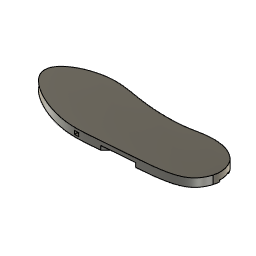
Smart foot brace v3 (Autodesk Fusion 360 design; units mm, degrees)
Autodesk Fusion 360 part; units mm, degrees
sketch "Schizzo2" plane through (0, 0, 0) normal (0, 0, 1) x (1, 0, 0)
  line L0 (-49.9969, 3.1408) -> (-49.9969, -77.002)
  line L1 (269.0032, -13.0421) -> (245.6537, -14.8322)
  line L2 (251.2577, -31.5554) -> (270.315, -30.0944)
  line L3 (270.315, -30.0944) -> (269.0032, -13.0421)
  spline S0 degree 5 poles (239.6431, -39.0842) (239.008, -40.9338) (237.6138, -44.5456) (235.154, -49.7023) (230.6516, -55.9329) (221.1905, -62.1637) (206.5229, -66.4683) (188.36, -69.1663) (168.6133, -70.9116) (148.4991, -72.3278) (128.8774, -73.8918) (110.0255, -75.6871) (91.7256, -77.2705) (73.0453, -77.351) (52.5897, -73.8128) (31.6095, -66.6537) (12.3777, -56.7145) (-2.2618, -45.4213) (-9.8521, -34.1339) (-8.9725, -23.6462) (-0.2666, -13.6017) (14.0848, -4.9823) (31.2393, 1.0769) (48.4813, 3.7209) (63.9221, 3.1001) (77.5489, 1.0443) (90.8033, -1.4303) (105.5547, -3.5848) (122.705, -4.9647) (142.1637, -5.3299) (159.3113, -4.3034) (172.1696, -2.1405) (182.8837, 0.235) (193.8253, 1.7835) (206.3024, 1.6151) (216.9338, -0.4964) (223.8154, -3.6611) (228.407, -6.7709) (231.3167, -9.1532) (232.7333, -10.4216) knots 0 0 0 0 0 0 0.028571 0.057143 0.085714 0.114286 0.142857 0.171429 0.2 0.228571 0.257143 0.285714 0.314286 0.342857 0.371429 0.4 0.428571 0.457143 0.485714 0.514286 0.542857 0.571429 0.6 0.628571 0.657143 0.685714 0.714286 0.742857 0.771429 0.8 0.828571 0.857143 0.885714 0.914286 0.942857 0.971429 1 1 1 1 1 1
  line L4 (247.2731, -16.8633) -> (232.013, -61.305)
  line L5 (235.4873, -58.3623) -> (184.5271, -71.6971)
  line L6 (112.4168, -77.0193) -> (57.595, -77.0134)
  line L7 (-8.4307, -44.1652) -> (-8.4277, -15.72)
  line L8 (26.8163, 3.1326) -> (81.9854, 3.1268)
  line L9 (104.9495, -5.3071) -> (173.0776, -4.7372)
  line L10 (173.2743, 1.9517) -> (226.7543, 0.991)
  line L11 (214.0903, 6.2711) -> (251.3764, -27.1143)
  spline S1 degree 5 poles (239.6431, -39.0842) (239.8525, -38.4743) (240.3443, -37.3331) (241.301, -35.8564) (242.9551, -34.3027) (245.4512, -32.8887) (247.6708, -32.1165) (249.4288, -31.7477) (250.6413, -31.6027) (251.2577, -31.5554) knots 0 0 0 0 0 0 0.2 0.4 0.6 0.8 1 1 1 1 1 1
  spline S2 degree 5 poles (232.7333, -10.4216) (233.164, -10.8072) (234.0487, -11.5321) (235.446, -12.4805) (237.4316, -13.4935) (240.0595, -14.3948) (242.2482, -14.8107) (243.9334, -14.9127) (245.0769, -14.8765) (245.6537, -14.8322) knots 0 0 0 0 0 0 0.2 0.4 0.6 0.8 1 1 1 1 1 1
  line L12 (-8.4292, -101.5202) -> (241.5708, -101.5202)
  line L13 (269.9236, -11.9686) -> (245.5773, -13.8352)
  spline S3 degree 3 poles (233.4004, -9.6766) (235.2721, -11.3525) (237.4456, -12.4757) (239.7715, -13.1715) (241.6374, -13.7297) (243.5687, -13.9891) (245.5773, -13.8352) knots 0 0 0 0 0.554866 0.554866 0.554866 1 1 1 1
  spline S4 degree 3 poles (240.5888, -39.4089) (239.2288, -43.3698) (237.586, -47.1235) (235.258, -50.5942) (233.0296, -53.9163) (230.1256, -56.9559) (226.1195, -59.5307) (222.5382, -61.8324) (218.0521, -63.7558) (212.7264, -65.3147) (204.0376, -67.858) (193.2175, -69.4408) (181.8239, -70.6189) (171.6726, -71.6685) (161.0707, -72.4189) (150.6531, -73.2094) (141.2105, -73.9259) (131.9202, -74.686) (122.8812, -75.4938) (114.5446, -76.2388) (106.4233, -77.0328) (98.2848, -77.5487) (90.3505, -78.0515) (82.3633, -78.2665) (73.9671, -77.5846) (66.6167, -76.9877) (58.9395, -75.6792) (51.1766, -73.6098) (41.5761, -71.0505) (31.86, -67.3391) (23.0777, -62.9007) (14.0271, -58.3266) (6.0213, -53.0215) (0.2781, -47.5919) (-4.7696, -42.8201) (-8.0755, -37.953) (-9.0908, -33.1359) (-9.8586, -29.4927) (-9.2793, -25.8888) (-7.517, -22.488) (-4.7337, -17.1171) (0.9259, -12.1616) (8.0905, -7.9878) (14.6953, -4.1401) (22.5473, -1.0036) (30.4783, 1.0609) (36.8948, 2.7312) (43.3496, 3.689) (49.4389, 4.0032) (55.9944, 4.3414) (62.1106, 3.9625) (67.845, 3.3046) (75.3924, 2.4387) (82.3167, 1.1103) (89.6988, -0.1009) (95.7767, -1.098) (102.2122, -2.0254) (109.3408, -2.7161) (114.6842, -3.2339) (120.4332, -3.6238) (126.4033, -3.8401) (133.1258, -4.0837) (140.0715, -4.0995) (146.4427, -3.8471) (151.9175, -3.6301) (156.9467, -3.2154) (161.4118, -2.663) (169.3887, -1.6762) (175.6132, -0.2481) (181.8504, 0.8561) (185.556, 1.5122) (189.2963, 2.0447) (193.2224, 2.3041) (198.2672, 2.6374) (203.5926, 2.5112) (208.4512, 1.8288) (213.3705, 1.1379) (217.7793, -0.1161) (221.6768, -1.8868) (226.0615, -3.8789) (229.8582, -6.505) (233.4004, -9.6766) knots 0 0 0 0 0.03616105 0.03616105 0.03616105 0.07077455 0.07077455 0.07077455 0.10171712 0.10171712 0.10171712 0.15219932 0.15219932 0.15219932 0.19717723 0.19717723 0.19717723 0.23794526 0.23794526 0.23794526 0.27554534 0.27554534 0.27554534 0.31220121 0.31220121 0.31220121 0.34429112 0.34429112 0.34429112 0.38397767 0.38397767 0.38397767 0.42487674 0.42487674 0.42487674 0.46082195 0.46082195 0.46082195 0.48800841 0.48800841 0.48800841 0.53094375 0.53094375 0.53094375 0.57052484 0.57052484 0.57052484 0.60254726 0.60254726 0.60254726 0.63702043 0.63702043 0.63702043 0.68239288 0.68239288 0.68239288 0.71974977 0.71974977 0.71974977 0.74775154 0.74775154 0.74775154 0.77928259 0.77928259 0.77928259 0.80637744 0.80637744 0.80637744 0.85478308 0.85478308 0.85478308 0.88354135 0.88354135 0.88354135 0.92049365 0.92049365 0.92049365 0.95790815 0.95790815 0.95790815 1 1 1 1
  spline S5 degree 3 poles (240.5888, -39.4089) (241.3059, -37.3208) (242.5674, -35.9265) (244.2133, -34.8517) (245.985, -33.6946) (248.1383, -32.9425) (250.4491, -32.6435) (250.7409, -32.6057) (251.0358, -32.5753) (251.3342, -32.5525) knots 0 0 0 0 0.452012 0.452012 0.452012 0.938578 0.938578 0.938578 1 1 1 1
  line L14 (251.3342, -32.5525) -> (271.3887, -31.015)
  line L15 (271.3887, -31.015) -> (269.9236, -11.9686)
  spline S6 degree 3 poles (243.4498, -40.3145) (243.442, -40.3374) (243.4341, -40.3603) (243.4262, -40.3832) (242.0634, -44.3523) (240.3996, -48.2035) (238.0265, -51.8462) (235.6744, -55.4566) (232.5576, -58.8379) (228.3332, -61.6662) (224.4374, -64.2746) (219.6477, -66.3777) (214.0375, -68.0553) (204.0845, -71.0316) (191.6967, -72.693) (178.8207, -73.9334) (168.6765, -74.9106) (158.2217, -75.637) (148.0073, -76.4198) (138.7072, -77.1325) (129.5865, -77.902) (120.6933, -78.7021) (112.4086, -79.4474) (104.2918, -80.2322) (96.0615, -80.6859) (88.7013, -81.0916) (81.1926, -81.2067) (73.3032, -80.5399) (65.6523, -79.8932) (57.6694, -78.4919) (49.6214, -76.2976) (39.5371, -73.5481) (29.3854, -69.5745) (20.2705, -64.8326) (11.3691, -60.2017) (3.5101, -54.8955) (-2.2653, -49.3107) (-6.7675, -44.9572) (-10.0656, -40.3962) (-11.5628, -35.5397) (-11.7947, -34.7875) (-11.9824, -34.0288) (-12.123, -33.2646) (-12.8162, -29.4949) (-12.2823, -25.6931) (-10.7144, -22.2104) (-8.3374, -16.9306) (-3.8076, -12.3656) (1.8783, -8.3928) (2.4386, -8.0013) (3.0106, -7.6156) (3.5933, -7.2357) (10.8043, -2.5345) (19.6906, 1.2501) (28.7492, 3.7056) (35.3784, 5.5025) (42.0699, 6.5654) (48.4105, 6.9501) (55.1171, 7.3571) (61.376, 7.0246) (67.1852, 6.3967) (74.9752, 5.5546) (82.0081, 4.2133) (89.3533, 2.9966) (95.368, 2.0003) (101.6744, 1.0688) (108.6597, 0.3657) (113.8765, -0.1593) (119.4922, -0.5623) (125.3539, -0.7978) (132.0277, -1.066) (138.9779, -1.1101) (145.3609, -0.8855) (150.7837, -0.6946) (155.782, -0.3097) (160.2056, 0.2129) (167.2628, 1.0468) (172.9356, 2.2385) (178.5539, 3.3007) (182.5227, 4.0511) (186.4973, 4.7256) (190.7246, 5.1154) (195.4849, 5.5543) (200.543, 5.6207) (205.4013, 5.1935) (210.2533, 4.7669) (214.8072, 3.8537) (218.9098, 2.4397) (225.3474, 0.2209) (230.6534, -3.1902) (235.4016, -7.4416) (235.428, -7.4652) (235.4544, -7.4889) (235.4808, -7.5125) knots -0.00020611 -0.00020611 -0.00020611 -0.00020611 0 0 0 0.03482635 0.03482635 0.03482635 0.06918618 0.06918618 0.06918618 0.10083869 0.10083869 0.10083869 0.15703627 0.15703627 0.15703627 0.20132062 0.20132062 0.20132062 0.24164672 0.24164672 0.24164672 0.27922087 0.27922087 0.27922087 0.31279914 0.31279914 0.31279914 0.34534649 0.34534649 0.34534649 0.38613373 0.38613373 0.38613373 0.4259753 0.4259753 0.4259753 0.45704046 0.45704046 0.45704046 0.46185185 0.46185185 0.46185185 0.4854789 0.4854789 0.4854789 0.52150819 0.52150819 0.52150819 0.52505893 0.52505893 0.52505893 0.56895312 0.56895312 0.56895312 0.60106672 0.60106672 0.60106672 0.63505887 0.63505887 0.63505887 0.68067651 0.68067651 0.68067651 0.71802793 0.71802793 0.71802793 0.74591886 0.74591886 0.74591886 0.777679 0.777679 0.777679 0.80466247 0.80466247 0.80466247 0.8477088 0.8477088 0.8477088 0.87807551 0.87807551 0.87807551 0.91224796 0.91224796 0.91224796 0.94637208 0.94637208 0.94637208 1 1 1 1.0003083 1.0003083 1.0003083 1.0003083
  arc A0 (243.4498, -40.3145) -> (235.4808, -7.5125) centre (209.2626, -31.2511) ccw
  point P0 (-8.4292, -29.9426)
  point P1 (54.4009, 3.1297)
  point P2 (139.0136, -5.0221)
  point P3 (200.0143, 1.4714)
  point P4 (85.0059, -77.0164)
  point P5 (210.0072, -65.0297)
  point P6 (85.0059, -77.0164)
  point P7 (85.0059, -81.0152)
  dimension "d6" = 80.1428
  dimension "d10" = 250
  dimension "d15" = 1
  constraint parallel L1 L2
  constraint midpoint S0.start L4
  constraint midpoint P5 L5
  constraint midpoint P6 L6
  constraint midpoint P0 L7
  constraint midpoint P1 L8
  constraint midpoint P2 L9
  constraint midpoint P3 L10
  constraint midpoint S0.end L11
  constraint horizontal L12
  constraint vertical L0
  constraint coincident P6 P4
  constraint coincident S6 P7
  measures "d6" distance of L0.start L0.end
  measures "d10" distance of L12.start L12.end
extrude "Estrusione3" add sketch "Schizzo2" against normal blind 12 contours L11 S2 A0 | L11 S2 S3 S4 A0 | S0 L4 L11 A0 | S0 L10 L11 S4 | L10 L11 S3 S4 S6 A0 | L4 S1 S4 S5 A0 | L4 S1 A0 | S0 L8 L10 S4 | L10 S4 | L10 L11 S4 | S0 L4 L5 S4 | L4 S4 S5 S6 A0 | L7 L10 L11 S4 S6 | L10 L11 S6 | S0 L5 L6 S4 | L5 S4 | L4 L5 S4 S6 | S0 L7 L8 S4 | L8 S4 | S0 L6 L7 S4 | L6 S4 | L5 L7 S4 S6 | L7 S4 | L7 S4 S6
extrude "Estrusione4" [suppressed]
ref_plane "Piano di lavoro1" through (85.0059, -81.0152, 0) normal (-0.000242, -1, 0) x (1, -0.000242, 0)
sketch "Schizzo5" plane through (85.0059, -81.0152, 0) normal (-0.000242, -1, 0) x (1, -0.000242, 0)
  line L0 (158.4341, -12) -> (-97.4394, -12)
  line L1 (-93.4302, 0) -> (156.5698, 0)
  line L2 (6.35, -9.7) -> (-6.35, -9.7)
  line L3 (-6.35, -9.7) -> (-6.35, -3)
  line L4 (-6.35, -3) -> (6.35, -3)
  line L5 (6.35, -3) -> (6.35, -9.7)
  line L6 (3, -8.85) -> (-3, -8.85)
  line L7 (-3, -8.85) -> (-3, -3.85)
  line L8 (-3, -3.85) -> (3, -3.85)
  line L9 (3, -3.85) -> (3, -8.85)
  point P0 (1, -1)
  dimension "d56" = 3
  dimension "d57" = 12.7
  dimension "d58" = 6.7
  dimension "d59" = 6
  dimension "d60" = 5
  dimension "d62" = 0.85
  dimension "d63" = 3.35
  constraint horizontal L2
  constraint vertical L3
  constraint horizontal L4
  constraint vertical L5
  constraint horizontal L6
  constraint vertical L7
  constraint horizontal L8
  constraint vertical L9
  measures "d56" distance of L1 L4
  measures "d57" distance of L3.end L4.end
  measures "d58" distance of L2.start L4.end
  measures "d59" distance of L6.start L6.end
  measures "d60" distance of L6 L8
  measures "d62" distance of L2 L6
  measures "d63" distance of L3 L7
extrude "Estrusione11" cut sketch "Schizzo5" against normal blind 18.5 contours L6 L7 L8 L9
extrude "Estrusione12" cut sketch "Schizzo5" against normal blind 14.5 from surface at -4
extrude "Estrusione13" cut 1 faces at (82.8925, -67.348, -3) along direction (0, 0, -1) blind 20
sketch "Schizzo3" plane through (0, 0, -12) normal (0, 0, -1) x (1, 0, 0)
  arc A0 (235.4808, 7.5125) -> (243.4498, 40.3145) centre (209.2626, 31.2511) ccw
  spline S0 degree 3 poles (243.4498, 40.3145) (243.442, 40.3374) (243.4341, 40.3603) (243.4262, 40.3832) (242.0634, 44.3523) (240.3996, 48.2035) (238.0265, 51.8462) (235.6744, 55.4566) (232.5576, 58.8379) (228.3332, 61.6662) (224.4374, 64.2746) (219.6477, 66.3777) (214.0375, 68.0553) (204.0845, 71.0316) (191.6967, 72.693) (178.8207, 73.9334) (168.6765, 74.9106) (158.2217, 75.637) (148.0073, 76.4198) (138.7072, 77.1325) (129.5865, 77.902) (120.6933, 78.7021) (112.4086, 79.4474) (104.2918, 80.2322) (96.0615, 80.6859) (88.7013, 81.0916) (81.1926, 81.2067) (73.3032, 80.5399) (65.6523, 79.8932) (57.6694, 78.4919) (49.6214, 76.2976) (39.5371, 73.5481) (29.3854, 69.5745) (20.2705, 64.8326) (11.3691, 60.2017) (3.5101, 54.8955) (-2.2653, 49.3107) (-6.7675, 44.9572) (-10.0656, 40.3962) (-11.5628, 35.5397) (-11.7947, 34.7875) (-11.9824, 34.0288) (-12.123, 33.2646) (-12.8162, 29.4949) (-12.2823, 25.6931) (-10.7144, 22.2104) (-8.3374, 16.9306) (-3.8076, 12.3656) (1.8783, 8.3928) (2.4386, 8.0013) (3.0106, 7.6156) (3.5933, 7.2357) (10.8043, 2.5345) (19.6906, -1.2501) (28.7492, -3.7056) (35.3784, -5.5025) (42.0699, -6.5654) (48.4105, -6.9501) (55.1171, -7.3571) (61.376, -7.0246) (67.1852, -6.3967) (74.9752, -5.5546) (82.0081, -4.2133) (89.3533, -2.9966) (95.368, -2.0003) (101.6744, -1.0688) (108.6597, -0.3657) (113.8765, 0.1593) (119.4922, 0.5623) (125.3539, 0.7978) (132.0277, 1.066) (138.9779, 1.1101) (145.3609, 0.8855) (150.7837, 0.6946) (155.782, 0.3097) (160.2056, -0.2129) (167.2628, -1.0468) (172.9356, -2.2385) (178.5539, -3.3007) (182.5227, -4.0511) (186.4973, -4.7256) (190.7246, -5.1154) (195.4849, -5.5543) (200.543, -5.6207) (205.4013, -5.1935) (210.2533, -4.7669) (214.8072, -3.8537) (218.9098, -2.4397) (225.3474, -0.2209) (230.6534, 3.1902) (235.4016, 7.4416) (235.428, 7.4652) (235.4544, 7.4889) (235.4808, 7.5125) knots -0.00020611 -0.00020611 -0.00020611 -0.00020611 0 0 0 0.03482635 0.03482635 0.03482635 0.06918618 0.06918618 0.06918618 0.10083869 0.10083869 0.10083869 0.15703627 0.15703627 0.15703627 0.20132062 0.20132062 0.20132062 0.24164672 0.24164672 0.24164672 0.27922087 0.27922087 0.27922087 0.31279914 0.31279914 0.31279914 0.34534649 0.34534649 0.34534649 0.38613373 0.38613373 0.38613373 0.4259753 0.4259753 0.4259753 0.45704046 0.45704046 0.45704046 0.46185185 0.46185185 0.46185185 0.4854789 0.4854789 0.4854789 0.52150819 0.52150819 0.52150819 0.52505893 0.52505893 0.52505893 0.56895312 0.56895312 0.56895312 0.60106672 0.60106672 0.60106672 0.63505887 0.63505887 0.63505887 0.68067651 0.68067651 0.68067651 0.71802793 0.71802793 0.71802793 0.74591886 0.74591886 0.74591886 0.777679 0.777679 0.777679 0.80466247 0.80466247 0.80466247 0.8477088 0.8477088 0.8477088 0.87807551 0.87807551 0.87807551 0.91224796 0.91224796 0.91224796 0.94637208 0.94637208 0.94637208 1 1 1 1.0003083 1.0003083 1.0003083 1.0003083
  line L0 (-9.0133, 39.7235) -> (19.2267, 39.7235)
  line L1 (19.2267, 39.7235) -> (19.2267, 20.4235)
  line L2 (19.2267, 20.4235) -> (-9.0133, 20.4235)
  line L3 (-9.0133, 20.4235) -> (-9.0133, 39.7235)
  line L4 (-1.0133, 25.8735) -> (-17.0133, 25.8735)
  line L5 (-17.0133, 25.8735) -> (-17.0133, 34.2735)
  line L6 (-17.0133, 34.2735) -> (-1.0133, 34.2735)
  line L7 (-1.0133, 34.2735) -> (-1.0133, 25.8735)
  line L8 (-1.0133, 25.8735) -> (-17.0133, 34.2735) construction
  line L9 (-17.0133, 25.8735) -> (-1.0133, 34.2735) construction
  line L10 (73.2267, 49.9714) -> (92.2267, 49.9714)
  line L11 (92.2267, 49.9714) -> (92.2267, 17.9714)
  line L12 (92.2267, 17.9714) -> (73.2267, 17.9714)
  line L13 (73.2267, 17.9714) -> (73.2267, 49.9714)
  line L14 (19.2267, 49.9714) -> (73.2267, 49.9714)
  line L15 (73.2267, 49.9714) -> (73.2267, 13.9714)
  line L16 (73.2267, 13.9714) -> (19.2267, 13.9714)
  line L17 (19.2267, 13.9714) -> (19.2267, 49.9714)
  line L18 (92.2267, 49.9714) -> (119.6267, 49.9714)
  line L19 (119.6267, 49.9714) -> (119.6267, 24.5714)
  line L20 (119.6267, 24.5714) -> (92.2267, 24.5714)
  line L21 (92.2267, 24.5714) -> (92.2267, 49.9714)
  line L22 (122.6267, 61.7471) -> (164.6267, 61.7471)
  line L23 (164.6267, 61.7471) -> (164.6267, 5.6113)
  line L24 (164.6267, 5.6113) -> (122.6267, 5.6113)
  line L25 (122.6267, 5.6113) -> (122.6267, 61.7471)
  line L26 (251.2577, 31.5554) -> (270.315, 30.0944)
  line L27 (270.315, 30.0944) -> (269.0032, 13.0421)
  line L28 (269.0032, 13.0421) -> (245.6537, 14.8322)
  line L29 (270.315, 30.0944) -> (269.0032, 13.0421)
  line L30 (269.0032, 13.0421) -> (209.18, 17.6439)
  line L31 (209.18, 17.6439) -> (210.4917, 34.6962)
  line L32 (210.4917, 34.6962) -> (270.315, 30.0944)
  line L33 (91.3569, 77.0167) -> (91.3604, 62.5167)
  line L34 (91.3604, 62.5167) -> (78.6604, 62.5136)
  line L35 (78.6604, 62.5136) -> (78.6569, 77.0136)
  line L36 (78.6569, 77.0136) -> (91.3569, 77.0167)
  line L37 (122.6267, 59.9714) -> (19.2267, 59.9714)
  line L38 (19.2267, 59.9714) -> (19.2267, 49.9714)
  line L39 (19.2267, 49.9714) -> (122.6267, 49.9714)
  line L40 (19.2267, 49.9714) -> (24.2267, 49.9714)
  line L41 (92.2267, 17.9714) -> (74.7267, 17.9714)
  line L42 (91.3604, 62.5167) -> (78.6619, 62.5167)
  line L43 (78.6619, 62.5167) -> (78.6619, 59.9714)
  line L44 (78.6619, 59.9714) -> (91.3604, 59.9714)
  line L45 (91.3604, 59.9714) -> (91.3604, 62.5167)
  line L46 (164.6267, 61.7471) -> (217.4262, 61.7471)
  line L47 (217.4262, 61.7471) -> (217.4262, 3.1169)
  line L48 (164.6267, 5.6113) -> (164.6267, 61.7471)
  spline S1 degree 5 poles (217.4262, 61.7471) (218.0377, 61.7142) (219.4226, 61.5343) (221.9857, 60.9195) (226.1571, 59.1373) (231.456, 53.9479) (235.4591, 45.0282) (236.9817, 32.4295) (235.4708, 19.7987) (231.4862, 10.8184) (226.2021, 5.5804) (222.0289, 3.8067) (219.4504, 3.2419) (218.0481, 3.1169) (217.4262, 3.1169) knots 0 0 0 0 0 0 0.1 0.2 0.3 0.4 0.5 0.6 0.7 0.8 0.9 1 1 1 1 1 1
  line L49 (219.644, 3.1169) -> (215.2084, 3.1169)
  line L50 (215.2084, 61.8666) -> (219.644, 61.6277)
  line L51 (236.2326, 42.3953) -> (236.2326, 22.3953)
  line L52 (164.6267, 5.6113) -> (217.4262, 3.1169)
  line L53 (19.2267, 49.9714) -> (19.2267, 39.7235)
  line L54 (19.2267, 20.4235) -> (19.2267, 5.6113)
  line L55 (19.2267, 5.6113) -> (122.6267, 5.6113)
  line L56 (54.1811, 49.9714) -> (38.2724, 49.9714)
  line L57 (38.2724, 49.9714) -> (38.2724, 52.9714)
  line L58 (38.2724, 52.9714) -> (54.1811, 52.9714)
  line L59 (54.1811, 52.9714) -> (54.1811, 49.9714)
  line L60 (38.2724, 13.9714) -> (54.1811, 13.9714)
  line L61 (54.1811, 13.9714) -> (54.1811, 10.9714)
  line L62 (54.1811, 10.9714) -> (38.2724, 10.9714)
  line L63 (38.2724, 10.9714) -> (38.2724, 13.9714)
  line L64 (73.2267, 14.9714) -> (76.2267, 14.9714)
  line L65 (76.2267, 14.9714) -> (76.2267, 17.9714)
  line L66 (92.2267, 21.5714) -> (98, 21.5714)
  line L67 (98, 21.5714) -> (98, 24.5714)
  line L68 (89.0639, 49.9714) -> (89.0639, 52.9714)
  line L69 (89.0639, 52.9714) -> (95.0639, 52.9714)
  line L70 (122.6267, 52.9714) -> (116.6267, 52.9714)
  line L71 (116.6267, 52.9714) -> (116.6267, 49.9714)
  line L72 (119.6267, 24.5714) -> (122.6267, 24.5714)
  line L73 (95.0639, 52.9714) -> (95.0639, 49.9714)
  line L74 (139.4267, 64.0107) -> (147.8267, 64.0107)
  line L75 (147.8267, 64.0107) -> (147.8267, 59.4836)
  line L76 (147.8267, 59.4836) -> (139.4267, 59.4836)
  line L77 (139.4267, 59.4836) -> (139.4267, 64.0107)
  line L78 (139.4267, 64.0107) -> (147.8267, 59.4836) construction
  line L79 (147.8267, 64.0107) -> (139.4267, 59.4836) construction
  line L80 (151.8267, 61.7471) -> (171.7987, 81.7191)
  line L81 (171.7987, 81.7191) -> (115.4547, 81.7191)
  line L82 (115.4547, 81.7191) -> (135.4267, 61.7471)
  point P0 (-9.0133, 30.0735)
  point P1 (244.6267, 30.6453)
  point P2 (247.758, 30.6453)
  point P3 (236.2326, 32.3953)
  point P4 (46.2267, 13.9714)
  point P5 (143.6267, 61.7471)
  point P6 (143.6267, 61.7471)
  dimension "d36" = 28.24
  dimension "d37" = 19.3
  dimension "d38" = 8.4
  dimension "d43" = 32
  dimension "d44" = 19
  dimension "d45" = 54
  dimension "d46" = 36
  dimension "d47" = 27.4
  dimension "d48" = 25.4
  dimension "d88" = 60
  dimension "d92" = 10
  dimension "d93" = 5
  dimension "d120" = 80
  dimension "d121" = 42
  dimension "d123" = 3
  dimension "d126" = 8
  dimension "d127" = 3
  dimension "d128" = 3
  dimension "d129" = 3
  dimension "d130" = 3
  dimension "d131" = 3
  dimension "d133" = 3
  dimension "d134" = 6
  dimension "d140" = 3
  dimension "d141" = 6
  dimension "d142" = 8.4
  dimension "d143" = 4
  dimension "d144" = 4
  dimension "d145" = 135
  dimension "d146" = 45
  constraint horizontal L0
  constraint vertical L1
  constraint horizontal L2
  constraint vertical L3
  constraint horizontal L4
  constraint perpendicular L4 L5
  constraint parallel L4 L6
  constraint parallel L5 L7
  constraint coincident L8 P0
  constraint coincident L9 P0
  constraint midpoint L3 P0
  constraint horizontal L10
  constraint vertical L11
  constraint horizontal L12
  constraint vertical L13
  constraint horizontal L14
  constraint vertical L15
  constraint horizontal L16
  constraint vertical L17
  constraint horizontal L18
  constraint vertical L19
  constraint horizontal L20
  constraint vertical L21
  constraint horizontal L22
  constraint vertical L23
  constraint horizontal L24
  constraint vertical L25
  constraint perpendicular L29 L30
  constraint parallel L29 L31
  constraint parallel L30 L32
  constraint coincident L27.end L28.start
  constraint parallel L27 L29
  constraint coincident L26.end L27.start
  constraint horizontal L37
  constraint vertical L38
  constraint horizontal L39
  constraint collinear L18 L39
  constraint collinear L10 L39
  constraint collinear L14 L39
  constraint collinear L1 L38
  constraint horizontal L40
  constraint horizontal L41
  constraint horizontal L42
  constraint vertical L43
  constraint horizontal L44
  constraint vertical L45
  constraint coincident L37 L43.end
  constraint coincident L33.end L34.start
  constraint coincident L25 L37.start
  constraint coincident L25 L39.end
  constraint coincident L22.start L25.end
  constraint horizontal L46
  constraint vertical L47
  constraint vertical L48
  constraint midpoint L47.end L49
  constraint midpoint L46.end L50
  constraint midpoint P3 L51
  constraint perpendicular L2 L54
  constraint horizontal L55
  constraint horizontal L56
  constraint vertical L57
  constraint horizontal L58
  constraint vertical L59
  constraint coincident L14 L56.start
  constraint coincident L39 L56.start
  constraint horizontal L60
  constraint vertical L61
  constraint horizontal L62
  constraint vertical L63
  constraint coincident L16 L60.start
  constraint collinear L59 L61
  constraint collinear L57 L63
  constraint midpoint L60 P4
  constraint midpoint L16 P4
  constraint coincident L15 L64.start
  constraint perpendicular L15 L64
  constraint coincident L41 L65.end
  constraint perpendicular L41 L65
  constraint coincident L11 L66.start
  constraint perpendicular L11 L66
  constraint coincident L20 L67.end
  constraint perpendicular L20 L67
  constraint coincident L10 L68.start
  constraint coincident L39 L68.start
  constraint perpendicular L10 L68
  constraint perpendicular L21 L69
  constraint coincident L25 L70.start
  constraint perpendicular L25 L70
  constraint coincident L18 L71.end
  constraint coincident L39 L71.end
  constraint vertical L71
  constraint coincident L25 L72.end
  constraint perpendicular L25 L72
  constraint collinear L17 L38
  constraint collinear L11 L21
  constraint collinear L13 L15
  constraint coincident L39 L73.end
  constraint vertical L73
  constraint midpoint L22 P6
  constraint horizontal L74
  constraint perpendicular L74 L75
  constraint parallel L74 L76
  constraint parallel L75 L77
  constraint coincident L78 P6
  constraint coincident L79 P6
  constraint coincident P6 P5
  constraint coincident L22 L80.start
  constraint coincident L22 L82.end
  constraint horizontal L81
  measures "d36" distance of L0.start L0.end
  measures "d37" distance of L0.start L2.end
  measures "d38" distance of L4.start L6.end
  measures "d43" distance of L10.end L11.end
  measures "d44" distance of L10.start L10.end
  measures "d45" distance of L14.start L10.start
  measures "d46" distance of L14.start L16.end
  measures "d47" distance of L10.end L18.end
  measures "d48" distance of L18.end L19.end
  measures "d88" distance of L26.end L31.end
  measures "d92" distance of L37.end L14.start
  measures "d93" distance of L14.start L40.end
  measures "d120" distance of L23 P1
  measures "d121" distance of L22.end L22.start
  measures "d123" distance of L19 L25
  measures "d126" distance of L3 L5
  measures "d127" distance of L60.end L61.end
  measures "d128" distance of L56.start L58.end
  measures "d129" distance of L64.end L65.end
  measures "d130" distance of L66.end L67.end
  measures "d131" distance of L68.start L68.end
  measures "d133" distance of L70.end L71.end
  measures "d134" distance of L70.start L70.end
  measures "d140" distance of L64.start L64.end
  measures "d141" distance of L68.end L69.end
  measures "d142" distance of L75.end L76.end
  measures "d143" distance of L75 L80.start
  measures "d144" distance of L77 L82.end
  measures "d145" angle of L22 L80
  measures "d146" angle of L22 L82
extrude "Estrusione21" cut sketch "Schizzo3" against normal blind 2 contours A0 L30 L32 S1 L51 | L30 L32 L47 S1 L51
extrude "Estrusione22" cut sketch "Schizzo3" against normal blind 6 contours L30 L47 S1 | L32 L47 S1 | L23 L30 L31 L32 L46 L47 L48 L52 | L30 L31 L32 L47 | S0 L22 L74 L75 L77 L80 L82 | L22 L23 L24 L25 L48 L75 L76 L77 | L22 L74 L75 L77 | L22 L75 L76 L77
extrude "Estrusione23" cut sketch "Schizzo3" against normal blind 8 contours L1 L13 L14 L15 L16 L17 L39 L40 L53 L54 L56 L60 | L11 L12 L15 L16 L20 L25 L41 L54 L55 L61 L62 L63 L64 L65 L66 L67 L72 | L19 L25 L39 L72 | L10 L14 L18 L25 L37 L38 L39 L40 L44 L57 L58 L59 L68 L69 L70 L71 L73 | L16 L60 L61 L62 L63 | L18 L25 L39 L70 L71 | L11 L18 L19 L20 L21 L39 | L34 L37 L42 L43 L44 L45 | L11 L20 L66 L67 | L14 L39 L56 L57 L58 L59 | L10 L11 L12 L13 L15 L21 L39 L41 | L12 L15 L41 L64 L65 | L10 L18 L39 L68 L69 L73
extrude "Estrusione24" cut sketch "Schizzo3" against normal blind 5 contours S0 L4 L5 L6 | S0 L3 L4 L6 | L0 L1 L2 L3 L4 L6 L7 L17 | L3 L4 L6 L7
draft "Sformo1" angle -54.1 neutral plane through (0, 0, 0) pull (0, 0, 1) 1 faces at (217.4262, -28.445, -7.3333)
fillet "Raccordo11" radius 13.499 1 edges at (122.6267, -32.7913, -6)
fillet "Raccordo12" radius 2.867 1 edges at (85.0111, -62.5152, -4)
fillet "Raccordo13" radius 1.369 1 edges at (19.2267, -30.0735, -7)
fillet "Raccordo14" radius 0.561 2 edges at (135.4267, -61.7471, -9) (151.8267, -61.7471, -9)
equation "MCU_w = 40 mm"
equation "MCU_l = 56 mm"
equation "MCU_h = 3 mm"
equation "Batt_l = 52 mm"
equation "Batt_w = 34 mm"
equation "Batt_h = 5 mm"
equation "ModRic_l = 28.5 mm"
equation "ModRic_w = 17.3 mm"
equation "ModRic_h = 5 mm"
equation "ModRic_l_onlyboard = 26.24 mm"
equation "IMU_w_l = 25.4 mm"
equation "IMU_h = 6 mm"
equation "Buck_l = 30 mm"
equation "Buck_w = 17 mm"
equation "Buck_h = 8 mm"
equation "d36 = ModRic_l_onlyboard + Hor_tol"
equation "d37 = ModRic_w + Hor_tol"
equation "d38 = USB_c_receptacle"
equation "USB_c_receptacle = 8.4 mm"
equation "d43 = Buck_l + Hor_tol"
equation "d44 = Buck_w + Hor_tol"
equation "d45 = Batt_l + Hor_tol"
equation "d46 = Batt_w + Hor_tol"
equation "d47 = IMU_w_l + Hor_tol"
equation "d48 = IMU_w_l"
equation "Sw_corpo_l = 12.7 mm"
equation "Sw_corpo_w = 6.7 mm"
equation "Sw_pulsante_l = 4 mm"
equation "Sw_pulsante_w = 4 mm"
equation "Sw_pulsante_scorrimento = 6 mm"
equation "d57 = Sw_corpo_l"
equation "d58 = Sw_corpo_w"
equation "d59 = Sw_pulsante_scorrimento"
equation "d62 = ( d58 - d60 ) / 2"
equation "d63 = ( d57 - d59 ) / 2"
equation "Sw_intero_l = 18.5 mm"
equation "d78 = -Sw_intero_l"
equation "d81 = -Sw_pulsante_l"
equation "d82 = -Sw_intero_l + Sw_pulsante_l"
equation "Hor_tol = 2 mm"
equation "d121 = MCU_w + Hor_tol"
equation "Spacers = 3 mm"
equation "d123 = Spacers"
equation "d127 = Spacers"
equation "d128 = Spacers"
equation "d129 = Spacers"
equation "d130 = Spacers"
equation "d131 = Spacers"
equation "d133 = Spacers"
equation "d134 = Spacers * 2"
equation "d140 = Spacers"
equation "d141 = Spacers * 2"
equation "d142 = USB_c_receptacle"
equation "d149 = -MCU_h * 2"
equation "d153 = -ModRic_h"
